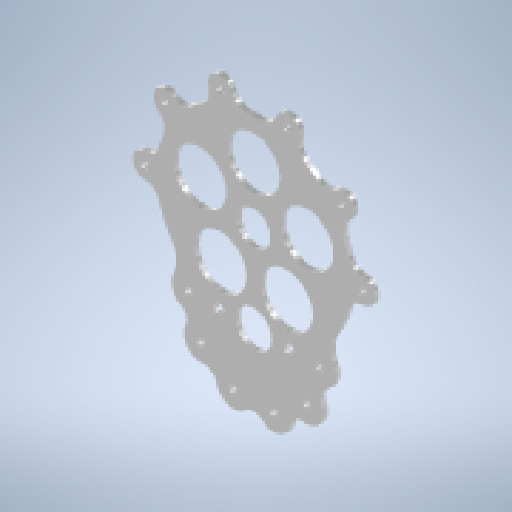
# Autodesk Inventor part: モーターマウント板
Saved by Autodesk Inventor 2024 (Build 280153000, 153)
## iProperties
Created: 2023-05-30
Part Number: モーターマウント板
Material: アルミニウム 6061
Document SubType Name: Modeling
Designer: yuta2
Density: 2.7 g/cm^3
Appearance: アルミニウム - フラット
Author: yuta2
Autodesk Inventor part; units mm, degrees
ref_plane "YZ Plane" through (0, 0, 0) normal (1, 0, 0) x (0, 1, 0)
ref_plane "XZ Plane" through (0, 0, 0) normal (0, 1, 0) x (-1, 0, 0)
ref_plane "XY Plane" through (0, 0, 0) normal (0, 0, 1) x (1, 0, 0)
sketch "スケッチ1" plane through (0, 0, 0) normal (0, 0, 1) x (1, 0, 0)
  circle A0 centre (0, 0) radius 40
  circle A1 centre (0, -36) radius 20
  point P0 (19.9555, -34.6667)
  point P1 (-19.9555, -34.6667)
  dimension "d0" = 80
  dimension "d1" = 40
  dimension "d2" = 36
  constraints: 2 centre point, 1 coincident, 1 vertical alignment
  measures "d0" diameter of A0
  measures "d1" diameter of A1
  measures "d2" distance of A1.centre A0.centre
extrude "押し出し1" add sketch "スケッチ1" along normal blind 2
sketch "スケッチ2" plane through (0, 0, 0) normal (0, 0, -1) x (-1, 0, 0)
  arc A0 (-19.9555, -34.6667) -> (19.9555, -34.6667) centre (0, -36) ccw projected
  point P0 (0, 0)
  constraints: 1 coincident
hole "穴1" at (0, -36, 0) direction (0, 0, 1) diameter 15 depth 4 tip angle 118
sketch "スケッチ3" plane through (0, 0, 0) normal (0, 0, -1) x (-1, 0, 0)
  circle A0 centre (0, -36) radius 7.5 projected
  arc A1 (-19.9555, -34.6667) -> (19.9555, -34.6667) centre (0, -36) ccw projected
  arc A2 (19.9555, -34.6667) -> (-19.9555, -34.6667) centre (0, 0) ccw projected
  circle A3 centre (0, -36) radius 7.5 projected
  point P0 (14.5, -36)
  point P1 (-14.5, -36)
  dimension "d12" = 14.5
  dimension "d13" = 14.5
  constraints: 2 horizontal alignment
  measures "d12" distance of A0.centre point (14.5, -36)
  measures "d13" distance of A3.centre point (-14.5, -36)
hole "穴2" at (-14.5, -36, 0) at (14.5, -36, 0) direction (0, 0, 1) diameter 4.1 depth 4 tip angle 118
sketch "スケッチ4" plane through (0, 0, 0) normal (0, 0, -1) x (-1, 0, 0)
  point P0 (0, 0)
  point P1 (0, 0)
  constraints: 1 coincident
hole "穴3" at (0, 0, 0) direction (0, 0, 1) diameter 14 depth 4 tip angle 118
sketch "スケッチ5" plane through (0, 0, 0) normal (0, 0, -1) x (-1, 0, 0)
  circle A0 centre (45, 0) radius 5
  arc A1 (19.9555, -34.6667) -> (-19.9555, -34.6667) centre (0, 0) ccw projected
  arc A2 (38.7692, 9.8462) -> (45, 5) centre (45, 11.4286) ccw
  arc A3 (19.9555, -34.6667) -> (-19.9555, -34.6667) centre (0, 0) ccw projected
  line L0 (0, 0) -> (40, 0)
  arc A4 (45, -5) -> (38.7692, -9.8462) centre (45, -11.4286) ccw
  point P0 (38.7692, -9.8462)
  point P1 (45, -5)
  dimension "d28" = 10
  constraints: 8 point on circle, 3 centre point, 3 symmetric about line, 3 tangent, 2 end point, 1 horizontal alignment, 1 vertical alignment, 1 other
  measures "d28" diameter of A0
extrude "押し出し2" add sketch "スケッチ5" against normal blind 2
pattern_circular "円形状パターン1" count 6 over 180 about axis through (0, 0, 0) along (0, 0, -1) of "押し出し2"
fillet "フィレット1" radius 5 2 edges at (-19.9555, -34.6667, 1) (19.9555, -34.6667, 1)
sketch "スケッチ6" plane through (0, 0, 0) normal (0, 0, -1) x (-1, 0, 0)
  circle A0 centre (0, 0) radius 7 projected
  circle A1 centre (-14.5, -36) radius 2.05 projected
  circle A2 centre (14.5, -36) radius 2.05 projected
  circle A3 centre (0, -36) radius 7.5 projected
  arc A4 (22.1851, -33.284) -> (19.9666, -37.1556) centre (24.9582, -37.4444) ccw projected
  arc A5 (22.1851, -33.284) -> (38.7692, -9.8462) centre (0, 0) ccw projected
  arc A6 (45, -5) -> (38.7692, -9.8462) centre (45, -11.4286) ccw projected
  arc A7 (45, -5) -> (45, 5) centre (45, 0) ccw projected
  arc A8 (38.7692, 9.8462) -> (45, 5) centre (45, 11.4286) ccw projected
  arc A9 (38.7692, 9.8462) -> (37.1524, 14.8223) centre (0, 0) ccw projected
  arc A10 (39.3447, 22.4053) -> (37.1524, 14.8223) centre (43.1233, 17.2044) ccw projected
  arc A11 (39.3447, 22.4053) -> (33.4668, 30.4954) centre (36.4058, 26.4503) ccw projected
  arc A12 (25.5775, 30.7537) -> (33.4668, 30.4954) centre (29.6882, 35.6962) ccw projected
  arc A13 (25.5775, 30.7537) -> (21.3446, 33.8291) centre (0, 0) ccw projected
  arc A14 (18.661, 41.2525) -> (21.3446, 33.8291) centre (24.775, 39.2659) ccw projected
  arc A15 (18.661, 41.2525) -> (9.1505, 44.3426) centre (13.9058, 42.7975) ccw projected
  arc A16 (2.6161, 39.9144) -> (9.1505, 44.3426) centre (3.0365, 46.3292) ccw projected
  arc A17 (2.6161, 39.9144) -> (-2.6161, 39.9144) centre (0, 0) ccw projected
  arc A18 (-9.1505, 44.3426) -> (-2.6161, 39.9144) centre (-3.0365, 46.3292) ccw projected
  arc A19 (-9.1505, 44.3426) -> (-18.661, 41.2525) centre (-13.9058, 42.7975) ccw projected
  arc A20 (-21.3446, 33.8291) -> (-18.661, 41.2525) centre (-24.775, 39.2659) ccw projected
  arc A21 (-21.3446, 33.8291) -> (-25.5775, 30.7537) centre (0, 0) ccw projected
  arc A22 (-33.4668, 30.4954) -> (-25.5775, 30.7537) centre (-29.6882, 35.6962) ccw projected
  arc A23 (-33.4668, 30.4954) -> (-39.3447, 22.4053) centre (-36.4058, 26.4503) ccw projected
  arc A24 (-37.1524, 14.8223) -> (-39.3447, 22.4053) centre (-43.1233, 17.2044) ccw projected
  arc A25 (-37.1524, 14.8223) -> (-38.7692, 9.8462) centre (0, 0) ccw projected
  arc A26 (-45, 5) -> (-38.7692, 9.8462) centre (-45, 11.4286) ccw projected
  arc A27 (-45, 5) -> (-45, -5) centre (-45, 0) ccw projected
  arc A28 (-38.7692, -9.8462) -> (-45, -5) centre (-45, -11.4286) ccw projected
  arc A29 (-38.7692, -9.8462) -> (-22.1851, -33.284) centre (0, 0) ccw projected
  arc A30 (-19.9666, -37.1556) -> (-22.1851, -33.284) centre (-24.9582, -37.4444) ccw projected
  arc A31 (-19.9666, -37.1556) -> (19.9666, -37.1556) centre (0, -36) ccw projected
  circle A32 centre (27, -36) radius 7
  arc A33 (-19.9666, -37.1556) -> (19.9666, -37.1556) centre (0, -36) ccw projected
  circle A34 centre (21.8435, -51.8702) radius 7
  circle A35 centre (8.3435, -61.6785) radius 7
  circle A36 centre (-8.3435, -61.6785) radius 7
  circle A37 centre (-21.8435, -51.8702) radius 7
  circle A38 centre (-27, -36) radius 7
  arc A39 (33.3913, -22.0232) -> (33.0691, -32.5119) centre (41.7391, -27.529) ccw
  arc A40 (22.1851, -33.284) -> (38.7692, -9.8462) centre (0, 0) ccw projected
  arc A41 (30.2809, -42.1835) -> (28.1323, -48.7961) centre (32.6244, -46.6003) ccw
  line L0 (0, 0) -> (0, -36)
  arc A42 (-33.0691, -32.5119) -> (-33.3913, -22.0232) centre (-41.7391, -27.529) ccw
  arc A43 (20.8632, -58.8012) -> (15.2382, -62.888) centre (20.163, -63.752) ccw
  arc A44 (3.4764, -66.7096) -> (-3.4764, -66.7096) centre (0, -70.3033) ccw
  arc A45 (-15.2382, -62.888) -> (-20.8632, -58.8012) centre (-20.163, -63.752) ccw
  arc A46 (-28.1323, -48.7961) -> (-30.2809, -42.1835) centre (-32.6244, -46.6003) ccw
  point P0 (-33.3913, -22.0232)
  point P1 (-30.2809, -42.1835)
  point P2 (-28.1323, -48.7961)
  point P3 (-20.8632, -58.8012)
  point P4 (-15.2382, -62.888)
  point P5 (-3.4764, -66.7096)
  point P6 (3.4764, -66.7096)
  point P7 (15.2382, -62.888)
  point P8 (20.8632, -58.8012)
  dimension "d36" = 14
  dimension "d39" = 180
  dimension "d41" = 10
  dimension "d42" = 5
  dimension "d45" = 144
  constraints: 17 point on circle, 12 centre point, 4 tangent, 3 symmetric about line, 2 end point, 1 horizontal alignment, 1 vertical, 33 other
  measures "d36" diameter of A32
  measures "d41" radius of A39
  measures "d42" radius of A41
extrude "押し出し3" add sketch "スケッチ6" against normal blind 2 contours A5 A32 A4 | A32 A41 A34 A31 A4 | A5 A39 A32 | A34 A43 A35 A31 | A34 | A35 A44 A36 A31 | A35 | A36 A45 A37 A31 | A36 | A37 A46 A38 A30 A31 | A37 | A38 A29 A30 | A42 A29 A38 picked at (27.6672, -38.9818) picked at (-27.6672, -38.9818)
sketch "スケッチ7" plane through (0, 0, 0) normal (0, 0, -1) x (-1, 0, 0)
  arc A0 (-45, 5) -> (-45, -5) centre (-45, 0) ccw projected
  arc A1 (-33.4668, 30.4954) -> (-39.3447, 22.4053) centre (-36.4058, 26.4503) ccw projected
  arc A2 (-9.1505, 44.3426) -> (-18.661, 41.2525) centre (-13.9058, 42.7975) ccw projected
  arc A3 (18.661, 41.2525) -> (9.1505, 44.3426) centre (13.9058, 42.7975) ccw projected
  arc A4 (39.3447, 22.4053) -> (33.4668, 30.4954) centre (36.4058, 26.4503) ccw projected
  arc A5 (45, -5) -> (45, 5) centre (45, 0) ccw projected
  arc A6 (30.2809, -42.1835) -> (33.0691, -32.5119) centre (27, -36) ccw projected
  arc A7 (20.8632, -58.8012) -> (28.1323, -48.7961) centre (21.8435, -51.8702) ccw projected
  arc A8 (3.4764, -66.7096) -> (15.2382, -62.888) centre (8.3435, -61.6785) ccw projected
  arc A9 (-15.2382, -62.888) -> (-3.4764, -66.7096) centre (-8.3435, -61.6785) ccw projected
  arc A10 (-28.1323, -48.7961) -> (-20.8632, -58.8012) centre (-21.8435, -51.8702) ccw projected
  arc A11 (-33.0691, -32.5119) -> (-30.2809, -42.1835) centre (-27, -36) ccw projected
  point P0 (0, 0)
  constraints: 12 coincident
hole "穴4" at (45, 0, 0) at (36.4058, 26.4503, 0) at (13.9058, 42.7975, 0) at (-13.9058, 42.7975, 0) at (-36.4058, 26.4503, 0) at (-45, 0, 0) at (-27, -36, 0) at (-21.8435, -51.8702, 0) at (-8.3435, -61.6785, 0) at (8.3435, -61.6785, 0) at (21.8435, -51.8702, 0) at (27, -36, 0) direction (0, 0, 1) diameter 3.2 end through all
sketch "スケッチ8" plane through (0, 0, 0) normal (0, 0, -1) x (-1, 0, 0)
  circle A0 centre (0, 0) radius 7 projected
  circle A1 centre (0, 0) radius 12.5
  circle A2 centre (0, 0) radius 40
  arc A3 (33.3913, -22.0232) -> (38.7692, -9.8462) centre (0, 0) ccw projected
  circle A4 centre (0, 0) radius 34
  circle A5 centre (-22.1121, 7.1846) radius 10.75
  circle A6 centre (-13.666, -18.8096) radius 10.75
  circle A7 centre (13.666, -18.8096) radius 10.75
  circle A8 centre (22.1121, 7.1846) radius 10.75
  circle A9 centre (0, 23.25) radius 10.75
  dimension "d56" = 25
  dimension "d57" = 6
  dimension "d60" = 360
  constraints: 8 centre point, 2 coincident, 2 tangent, 1 concentric, 1 horizontal alignment, 11 other
  measures "d56" diameter of A1
  measures "d57" radial gap between concentric circles of A2 A4
extrude "押し出し4" cut sketch "スケッチ8" against normal through all contours A8 | A7 | A9 | A6 | A5
equation "\"d13\" = d12"
